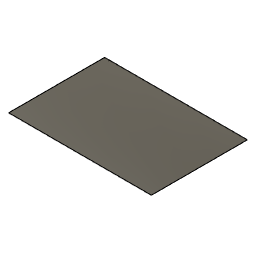
Lid v10 v3 (Autodesk Fusion 360 design; units mm, degrees)
Autodesk Fusion 360 part; units mm, degrees
sketch "LED window" plane through (0, 0, 0) normal (0, 0, 1) x (1, 0, 0)
  line L0 (23.6586, 17.7446) -> (-28.2697, 17.7446)
  line L1 (-28.2697, 17.7446) -> (-28.2697, -2.7419)
  line L2 (-28.2697, -2.7419) -> (23.6586, -2.7419)
  line L3 (23.6586, -2.7419) -> (23.6586, 17.7446)
  constraint horizontal L0
  constraint vertical L1
  constraint horizontal L2
  constraint vertical L3
sketch "Bottom" plane through (0, 0, 0) normal (0, 0, 1) x (1, 0, 0)
  line L0 (-37.1804, -23.3607) -> (36.4196, -23.3607)
  line L1 (36.4196, -23.3607) -> (36.4196, 26.1393)
  line L2 (36.4196, 26.1393) -> (-37.1804, 26.1393)
  line L3 (-37.1804, 26.1393) -> (-37.1804, -23.3607)
  dimension "d148" = 73.6
  dimension "d149" = 49.5
  constraint horizontal L0
  constraint vertical L1
  constraint horizontal L2
  constraint vertical L3
  measures "d148" distance of L0.start L0.end
  measures "d149" distance of L0.start L2.end
extrude "Extrude32" add sketch "Bottom" along normal blind 1.5 draft -45 makes body 1
ref_plane "WorkPlane3" through (-37.1804, 1.3893, 0) normal (1, 0, 0) x (0, -1, 0)
sketch "Sketch23" plane through (-37.1804, -58.3607, 0) normal (1, 0, 0) x (0, 1, 0)
  line L0 (84.5, 0) -> (35, 0)
  line L1 (35, 0) -> (35, 1.5002)
  line L2 (35, 1.5002) -> (84.5, 1.5002)
  line L3 (84.5, 1.5002) -> (84.5, 0)
  line L4 (35, 0) -> (36.5005, 1.5002)
  line L5 (82.9998, 1.5002) -> (84.5, 1.5002)
  line L6 (82.9998, 1.5002) -> (84.5, 0)
  line L7 (84.5, 0) -> (84.5, 1.5002)
  point P0 (84.5, 0)
  dimension "d167" = 49.5
  constraint horizontal L0
  constraint vertical L1
  constraint vertical L3
  constraint coincident P0 L0.start
  constraint coincident L2 L4.end
  constraint coincident L2 L5.start
  constraint perpendicular L5 L7
  measures "d167" distance of P0 L0.end
extrude "Extrude33" add sketch "Sketch23" along normal blind 1 contours L0 L2 L4 L6 bodies 1
extrude "Extrude34" add 1 faces at (-36.1804, -6.3605, 1.1667) along direction (1, 0, 0) blind 1.4 on bodies 1 bodies 1
mirror "Mirror1" about plane through (0, 0, 0) normal (0, 0, 1) of bodies 1 makes body 2
hidden bodies 1
equation "WINDOW_H = 7 mm"
equation "WINDOW_W = 4 mm"
equation "TOP_H = 1.5 mm"
equation "WALL = 18.5 mm + TOP_H"
equation "TOP_Z = 75.5 mm"
equation "TOP_HEIGHT = 52 mm"
equation "TOP_WIDTH = 75.5 mm"
equation "WALL_THICK = TOP_H"
equation "OUTER_DIAM = 4 mm"
equation "INNER_DIAM = 2.5 mm"
equation "CIRCLE_X_OFFSET = 41 mm"
equation "OUTER_HEIGHT = 6.4 mm + TOP_H"
equation "INNER_HEIGHT = OUTER_HEIGHT + 3.5 mm"
equation "d148 = TOP_WIDTH - ( WALL_THICK * 2 ) + 1.1 mm"
equation "d149 = TOP_HEIGHT - WALL_THICK * 2 - 0.5 mm"
equation "d150 = WALL_THICK"
equation "d167 = TOP_HEIGHT - WALL_THICK * 2 - 0.5 mm"
named bodies: "Lid", "Mirror"
